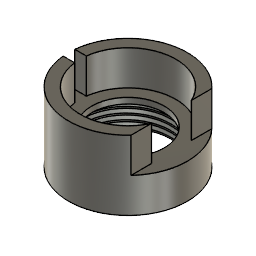
Lenshouder schroefdraad (Autodesk Fusion 360 design; units mm, degrees)
part number: 2026-06-04-13-28-36-774
Autodesk Fusion 360 part; units mm, degrees
sketch "Sketch2" plane through (0, 0, 0) normal (0, 0, 1) x (1, 0, 0)
  circle A0 centre (0, 0) radius 15
  dimension "d8" = 30
  constraint coincident A0.centre origin
  measures "d8" diameter of A0
extrude "Extrude3" add sketch "Sketch2" along normal blind 10 thin wall 5.5 outside makes body 1
sketch "Sketch1" plane through (0, 0, 10) normal (0, 0, 1) x (1, 0, 0)
  circle A0 centre (0, 0) radius 16.5
  circle A1 centre (0, 0) radius 15
  circle A2 centre (0, 0) radius 20.5
  dimension "d1" = 33
  constraint coincident A0.centre A1.centre
  measures "d1" diameter of A0
extrude "Extrude1" add sketch "Sketch1" along normal blind 14 thin wall 4 outside separate body contours A0 | A1 makes body 2
extrude "Extrude2" add sketch "Sketch1" along normal blind 2 thin wall 4 inside contours A0 | A1 bodies 2
sketch "Sketch3" plane through (0, 0, 24) normal (0, 0, 1) x (-1, 0, 0)
  circle A0 centre (0, 0) radius 16.5
  circle A1 centre (0, 0) radius 20.5
  line L0 (-21, 20) -> (-15, 20)
  line L1 (-15, 20) -> (-15, -20)
  line L2 (-15, -20) -> (-21, -20)
  line L3 (-21, -20) -> (-21, 20)
  line L4 (-21, 20) -> (-15, -20) construction
  line L5 (-15, 20) -> (-21, -20) construction
  line L6 (15.5, 2) -> (21.5, 2)
  line L7 (21.5, 2) -> (21.5, -2)
  line L8 (21.5, -2) -> (15.5, -2)
  line L9 (15.5, -2) -> (15.5, 2)
  line L10 (15.5, 2) -> (21.5, -2) construction
  line L11 (21.5, 2) -> (15.5, -2) construction
  point P0 (-18, 0)
  point P1 (18.5, 0)
  dimension "d12" = 6
  dimension "d13" = 40
  dimension "d16" = 15
  dimension "d17" = 20
  dimension "d18" = 6
  dimension "d19" = 4
  dimension "d20" = 15.5
  dimension "d21" = 2
  constraint horizontal L0
  constraint perpendicular L0 L1
  constraint parallel L0 L2
  constraint parallel L1 L3
  constraint coincident L4 P0
  constraint coincident L5 P0
  constraint horizontal L6
  constraint perpendicular L6 L7
  constraint parallel L6 L8
  constraint parallel L7 L9
  constraint coincident L10 P1
  constraint coincident L11 P1
  measures "d12" distance of L1.end L2.end
  measures "d13" distance of L0.end L1.end
  measures "d16" distance of A0.centre L1
  measures "d17" distance of A0.centre L2
  measures "d18" distance of L7.end L8.end
  measures "d19" distance of L6.end L7.end
  measures "d20" distance of A0.centre L9
  measures "d21" distance of A0.centre L8
extrude "Extrude4" cut sketch "Sketch3" against normal blind 12 contours A0 A1 L6 L8 | A0 A1 L1 bodies 2
thread "Thread1" "ISO Metric profile 32.0 M32x2 M32x2 6H" major diameter 32.2565 minor diameter 30.0224 pitch 2 angle 60 modelled right hand crest width 0.5434 on face at (14.9814, -0.7477, 6.6667) crest through (15.0112, 0, 0.5) on bodies 1
combine "Combine1" operation add target body 2 tool bodies 1
scale "Scale2" factor 1.008 about (-20.5, 0, 0) bodies 2
